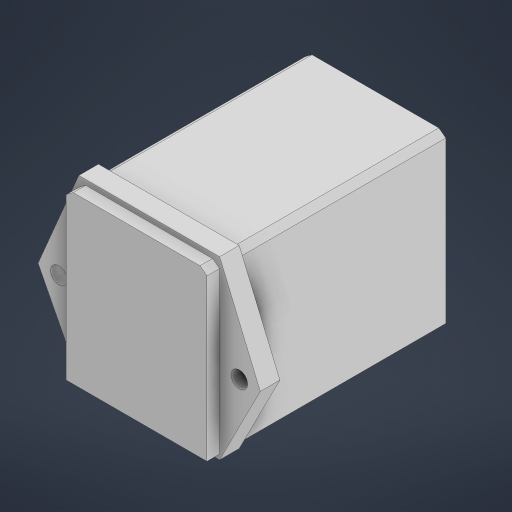
# Autodesk Inventor part: outlet
Saved by Autodesk Inventor 2024 (Build 280153000, 153)
## iProperties
Created: 2023-07-11
Part Number: outlet
Material: 일반
Document SubType Name: Modeling
Designer: 6gioc
Density: 1 g/cm^3
Appearance: 기본값
Author: 6gioc
Autodesk Inventor part; units mm, degrees
ref_plane "YZ Plane" through (0, 0, 0) normal (1, 0, 0) x (0, 1, 0)
ref_plane "XZ Plane" through (0, 0, 0) normal (0, 1, 0) x (-1, 0, 0)
ref_plane "XY Plane" through (0, 0, 0) normal (0, 0, 1) x (1, 0, 0)
sketch "스케치1" plane through (0, 0, 0) normal (0, 0, 1) x (1, 0, 0)
  line L0 (0, 0) -> (28, 0)
  line L1 (28, 0) -> (28, 33)
  line L2 (28, 33) -> (0, 33)
  line L3 (0, 33) -> (0, 0)
  line L4 (0, 34) -> (28, 34)
  line L5 (28, 34) -> (28, -1)
  line L6 (28, -1) -> (0, -1)
  line L7 (0, -1) -> (0, 34)
  circle A0 centre (-3.95, 14.85) radius 1.65
  circle A1 centre (31.95, 14.85) radius 1.65
  circle A2 centre (14, 14.85) radius 22.1
  line L8 (0, 34) -> (-8.1, 14.85)
  line L9 (-8.1, 14.85) -> (0, -1)
  line L10 (28, -1) -> (36.1, 14.85)
  line L11 (36.1, 14.85) -> (28, 34)
  point P0 (29.3923, 30.7084)
  point P1 (26.609, 33)
  point P2 (1.391, 33)
  point P3 (-1.3923, 30.7084)
  point P4 (0, 31.95)
  point P5 (28, 31.95)
  dimension "d0" = 28
  dimension "d1" = 33
  dimension "d2" = 28
  dimension "d3" = 35
  dimension "d4" = 1
  dimension "d5" = 3.3
  dimension "d6" = 3.3
  dimension "d7" = 35.9
  dimension "d8" = 3.95
  dimension "d9" = 15.85
  dimension "d10" = 44.2
  constraints: 24 end point, 4 parallel, 3 centre point, 2 horizontal, 2 perpendicular, 2 point on circle, 1 horizontal alignment, 1 point on line
  measures "d0" distance of L2.end L1.end
  measures "d1" distance of L1.end L0.end
  measures "d2" distance of L5.end L6.end
  measures "d3" distance of L4.end L5.end
  measures "d4" distance between parallel lines of L2 L4
  measures "d5" diameter of A0
  measures "d6" diameter of A1
  measures "d7" distance of A1.centre A0.centre
  measures "d8" distance from line of L3 A0.centre
  measures "d9" distance from line of L6 A0.centre
  measures "d10" diameter of A2
extrude "돌출1" add sketch "스케치1" against normal blind 3.9 contours L3 A2 L2 L1 L0 | L7 L9 L8 A2 L3 | L0 L5 L6 L7 | L1 A2 L11 L10 L5 | A2 L8 L7 L3 | L3 L2 A2 | A2 L2 L1 | L1 L5 L11 A2 | L7 L4 A2 L2 | A2 L4 L2 | L2 A2 L4 L5
extrude "돌출2" add sketch "스케치1" against normal blind 45 contours L3 A2 L2 L1 L0
extrude "돌출3" add sketch "스케치1" along normal blind 2.5 contours L3 A2 L2 L1 L0
